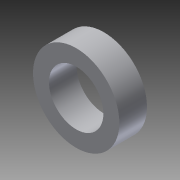
# Autodesk Inventor part: Spacer (0.4375 ID whatever OD) aluminum
Saved by Autodesk Inventor 2014 (Build 180170000, 170)
## iProperties
Created: 2014-01-20
Part Number: Spacer (0.4375 ID whatever OD) aluminum
Material: Aluminum 6061
Document SubType Name: Modeling
Designer: Andrew Toennies
Mass: 0.653976 g
Surface Area: 6.67429 cm^2
Volume: 0.241319 cm^3
Density: 2.71 g/cm^3
Appearance: Aluminum - Flat
Description: 92510A363
Author: Andrew Toennies
Autodesk Inventor part; units mm, degrees
ref_plane "YZ Plane" through (0, 0, 0) normal (1, 0, 0) x (0, 1, 0)
ref_plane "XZ Plane" through (0, 0, 0) normal (0, 1, 0) x (-1, 0, 0)
ref_plane "XY Plane" through (0, 0, 0) normal (0, 0, 1) x (1, 0, 0)
sketch "Sketch1" plane through (0, 0, 0) normal (0, 0, 1) x (1, 0, 0)
  circle A0 centre (0, 0) radius 8.001
  circle A1 centre (0, 0) radius 12.7
  line L0 (-2.6182, 14.4291) -> (11.1868, 9.482)
  line L1 (11.1868, 9.482) -> (13.8051, -4.9471)
  line L2 (13.8051, -4.9471) -> (2.6182, -14.4291)
  line L3 (2.6182, -14.4291) -> (-11.1868, -9.482)
  line L4 (-11.1868, -9.482) -> (-13.8051, 4.9471)
  line L5 (-13.8051, 4.9471) -> (-2.6182, 14.4291)
  point P0 (-8.2116, 9.6881)
  dimension "d1" = 25.4
  dimension "d0" = 16.002
  constraints: 12 end point, 3 coincident, 1 centre point, 1 midpoint, 16 other
  measures "d0" diameter of A0
extrude "Extrusion1" add sketch "Sketch1" along normal blind 8.128 contours A1
body "Solid1"
